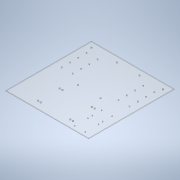
# Autodesk Inventor part: Electronics Base Plate
Saved by Autodesk Inventor 2022 (Build 260153000, 153)
## iProperties
Created: 2022-01-14
Part Number: Electronics Base Plate
Material: Generic
Document SubType Name: Modeling
Designer: merky
Density: 1 g/cm^3
Appearance: Polycarbonate - Clear
Author: merky
Autodesk Inventor part; units mm, degrees
ref_plane "YZ Plane" through (0, 0, 0) normal (1, 0, 0) x (0, 1, 0)
ref_plane "XZ Plane" through (0, 0, 0) normal (0, 1, 0) x (-1, 0, 0)
ref_plane "Work Plane1" through (0, 3.175, 0) normal (0, 1, 0) x (1, 0, 0)
sketch "Sketch2" plane through (0, 3.175, 0) normal (0, 1, 0) x (1, 0, 0)
  circle A0 centre (-82.55, 79.375) radius 1.8387
  circle A1 centre (-82.55, 142.875) radius 1.905
  circle A2 centre (-84.455, 336.55) radius 2.2218
  circle A3 centre (-238.125, 368.3) radius 2.667
  circle A4 centre (-346.075, 336.55) radius 2.2218
  circle A5 centre (-254, 133.35) radius 3.175
  circle A6 centre (-266.7, 133.35) radius 3.175
  line L0 (0, 393.7) -> (-381, 393.7)
  line L1 (-381, 393.7) -> (-381, 0)
  line L2 (-381, 0) -> (0, 0)
  line L3 (0, 0) -> (0, 393.7)
  line L4 (-381, 393.7) -> (-381, 0) projected
  line L5 (-381, 0) -> (0, 0) projected
  line L6 (-119.0443, 33.9146) -> (-119.0443, 186.178) construction
  circle A7 centre (-355.6, 368.3) radius 3.175
  circle A8 centre (-25.4, 368.3) radius 3.175
  circle A9 centre (-295.275, 336.55) radius 2.2218
  circle A10 centre (-346.075, 298.45) radius 2.2218
  circle A11 centre (-295.275, 298.45) radius 2.2218
  circle A12 centre (-346.075, 260.35) radius 2.2218
  circle A13 centre (-295.275, 260.35) radius 2.2218
  circle A14 centre (-346.075, 222.25) radius 2.2218
  circle A15 centre (-295.275, 222.25) radius 2.2218
  circle A16 centre (-33.655, 336.55) radius 2.2218
  circle A17 centre (-84.455, 298.45) radius 2.2218
  circle A18 centre (-33.655, 298.45) radius 2.2218
  circle A19 centre (-84.455, 260.35) radius 2.2218
  circle A20 centre (-33.655, 260.35) radius 2.2218
  circle A21 centre (-84.455, 222.25) radius 2.2218
  circle A22 centre (-33.655, 222.25) radius 2.2218
  circle A23 centre (-133.731, 368.3) radius 2.667
  circle A24 centre (-238.125, 188.8236) radius 2.667
  circle A25 centre (-133.731, 188.8236) radius 2.667
  circle A26 centre (-118.364, 133.35) radius 3.175
  circle A27 centre (-105.664, 133.35) radius 3.175
  circle A28 centre (-266.7, 33.909) radius 3.175
  circle A29 centre (-254, 33.909) radius 3.175
  circle A30 centre (-118.364, 33.909) radius 3.175
  circle A31 centre (-105.664, 33.909) radius 3.175
  circle A32 centre (-82.55, 18.3388) radius 1.8387
  circle A33 centre (-33.7058, 79.375) radius 1.8387
  circle A34 centre (-33.7058, 18.3388) radius 1.8387
  circle A35 centre (-82.55, 99.822) radius 1.905
  circle A36 centre (-34.798, 142.875) radius 1.905
  circle A37 centre (-34.798, 99.822) radius 1.905
  dimension "d19" = 6.35
  dimension "d20" = 6.35
  dimension "d21" = 12.7
  dimension "d40" = 6.35
  dimension "d41" = 25.4
  dimension "d42" = 25.4
  dimension "d43" = 6.35
  dimension "d44" = 25.4
  dimension "d45" = 25.4
  dimension "d51" = 57.15
  dimension "d52" = 34.925
  dimension "d53" = 4.4436
  dimension "d56" = 50.8
  dimension "d59" = 38.1
  dimension "d62" = 57.15
  dimension "d63" = 84.455
  dimension "d64" = 4.4436
  dimension "d67" = 50.8
  dimension "d70" = 38.1
  dimension "d73" = 25.4
  dimension "d74" = 142.875
  dimension "d79" = 104.394
  dimension "d82" = 179.4764
  dimension "d85" = 5.334
  dimension "d86" = 114.3
  dimension "d87" = 127
  dimension "d88" = 133.35
  dimension "d93" = 148.336
  dimension "d96" = 99.441
  dimension "d99" = 142.875
  dimension "d100" = 79.375
  dimension "d107" = 61.0362
  dimension "d110" = 48.8442
  dimension "d115" = 43.053
  dimension "d118" = 47.752
  dimension "d121" = 3.81
  dimension "d122" = 3.6774
  dimension "d123" = 3.6774
  dimension "d124" = 82.55
  dimension "d125" = 82.55
  constraints: 38 centre point, 10 end point, 9 vertical, 8 horizontal, 58 other
  measures "d19" diameter of A6
  measures "d20" diameter of A5
  measures "d21" distance of A6.centre A5.centre
  measures "d40" diameter of A7
  measures "d41" distance from line of L0 A7.centre
  measures "d42" distance from line of L4 A7.centre
  measures "d43" diameter of A8
  measures "d44" distance from line of A8.centre L3
  measures "d45" distance from line of A8.centre L0
  measures "d51" distance from line of L0 A4.centre
  measures "d52" distance from line of L4 A4.centre
  measures "d53" diameter of A4
  measures "d56" distance of A4.centre A9.centre
  measures "d59" distance of A4.centre A10.centre
  measures "d62" distance from line of L0 A2.centre
  measures "d63" distance from line of L3 A2.centre
  measures "d64" diameter of A2
  measures "d67" distance of A2.centre A16.centre
  measures "d70" distance of A2.centre A17.centre
  measures "d73" distance from line of L0 A3.centre
  measures "d74" distance from line of L1 A3.centre
  measures "d79" distance of A3.centre A23.centre
  measures "d82" distance of A3.centre A24.centre
  measures "d85" diameter of A23
  measures "d86" distance from line of L4 A6.centre
  measures "d87" distance from line of L4 A5.centre
  measures "d88" distance from line of L2 A5.centre
  measures "d93" distance of A6.centre A26.centre
  measures "d96" distance of A6.centre A28.centre
  measures "d99" distance from line of L2 A1.centre
  measures "d100" distance from line of L5 A0.centre
  measures "d107" distance of A0.centre A32.centre
  measures "d110" distance of A0.centre A33.centre
  measures "d115" distance of A1.centre A35.centre
  measures "d118" distance of A1.centre A36.centre
  measures "d121" diameter of A37
  measures "d122" diameter of A33
  measures "d123" diameter of A0
  measures "d124" distance from line of L3 A0.centre
  measures "d125" distance from line of L3 A1.centre
extrude "Extrusion3" add sketch "Sketch2" along normal blind 3.175
body "Solid1"
